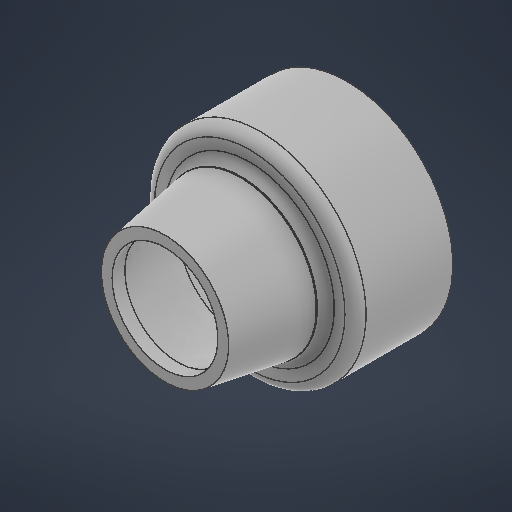
# Autodesk Inventor part: NOZZLE-EXTRUSOR
Saved by Autodesk Inventor 2025.3 (Build 293356030, 356C)
## iProperties
Created: 2025-09-01
Part Number: NOZZLE-EXTRUSOR
Material: Generic
Document SubType Name: Modeling
Designer: lstk1ng
Density: 1 g/cm^3
Appearance: Smooth - Medium Gray
Author: lstk1ng
Autodesk Inventor part; units mm, degrees
ref_plane "YZ Plane" through (0, 0, 0) normal (1, 0, 0) x (0, 1, 0)
ref_plane "XZ Plane" through (0, 0, 0) normal (0, 1, 0) x (-1, 0, 0)
ref_plane "XY Plane" through (0, 0, 0) normal (0, 0, 1) x (1, 0, 0)
sketch "Sketch1" plane through (0, 0, 0) normal (0, 1, 0) x (-1, 0, 0)
  line L0 (0, -11.9189) -> (0, 17.2618)
  line L1 (22, -8.4189) -> (22, 10.0811)
  line L2 (15, 15.0811) -> (15, 12.5811)
  line L3 (22, 10.0811) -> (17.5, 10.0811)
  line L4 (15, 15.0811) -> (12.5, 30.0811)
  line L5 (12.5, 33.0811) -> (15.0414, 33.0811)
  line L6 (15.0414, 33.0811) -> (18, 15.3294)
  line L7 (18, 15.3294) -> (18, 15.0811)
  line L8 (20, 13.0811) -> (22.5, 13.0811)
  line L9 (25, 10.5811) -> (25, -9.9189)
  line L10 (25, -9.9189) -> (23.5, -9.9189)
  line L11 (12.5, 30.0811) -> (12.5, 33.0811)
  line L12 (17.5, 10.0811) -> (15, 12.5811)
  arc A0 (25, 10.5811) -> (22.5, 13.0811) centre (22.5, 10.5811) ccw
  arc A1 (18, 15.0811) -> (20, 13.0811) centre (20, 15.0811) ccw
  line L13 (23.5, -9.9189) -> (22, -8.4189)
  point P0 (0, 0)
  point P1 (22, -9.9189)
  point P2 (15, 30.0811)
  point P3 (15, 10.0811)
  dimension "d14" = 20
  dimension "d15" = 44
  dimension "d22" = 15
  dimension "d23" = 2.5
  dimension "d24" = 2.5
  dimension "d25" = 2.5
  dimension "d26" = 2.5
  dimension "d27" = 2
  dimension "d28" = 1.5
  dimension "d29" = 1.5
  constraints: 28 end point, 5 point on line, 4 point on circle, 4 tangent, 2 centre point, 2 horizontal, 2 vertical, 1 perpendicular
  measures "d14" distance of point (22, -9.919) L1.end
  measures "d15" diameter of L1 L0
  measures "d22" distance of L2.start point (15, 30.081)
  measures "d23" distance of L4.end point (15, 30.081)
  measures "d24" distance of L3.end point (15, 10.081)
  measures "d25" distance of L2.end point (15, 10.081)
  measures "d26" radius of A0
  measures "d27" radius of A1
  measures "d28" distance of L10.end point (22, -9.919)
  measures "d29" distance of L1.start point (22, -9.919)
revolve "Revolution1" add sketch "Sketch1" angle 360 about axis through (0, 0, -11.9189) along (0, 0, 1)
equation "\"d25\" = d24"
equation "\"d29\" = d28"
body "Solid1"
